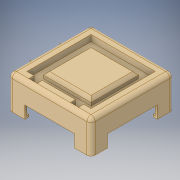
# Autodesk Inventor part: model for case
Saved by Autodesk Inventor 2016 (Build 200138000, 138)
## iProperties
Created: 2016-08-06
Part Number: model for case
Material: Polyethylene, High Density
Document SubType Name: Modeling
Designer: Jorian Brusind
Density: 0.952 g/cm^3
Appearance: Smooth - Off-White
Author: Jorian Brusind
Autodesk Inventor part; units mm, degrees
ref_plane "YZ Plane" through (0, 0, 0) normal (1, 0, 0) x (0, 1, 0)
ref_plane "XZ Plane" through (0, 0, 0) normal (0, 1, 0) x (-1, 0, 0)
ref_plane "XY Plane" through (0, 0, 0) normal (0, 0, 1) x (1, 0, 0)
sketch "Sketch4" plane through (0, 0, 0) normal (0, 1, 0) x (-1, 0, 0)
  line L0 (0, 0) -> (127, 0)
  line L1 (127, 0) -> (127, -127)
  line L2 (127, -127) -> (0, -127)
  line L3 (0, -127) -> (0, 0)
  dimension "d16" = 127
  dimension "d17" = 127
  constraints: 8 end point, 2 parallel, 1 horizontal, 1 perpendicular
  measures "d16" distance of L1.end L2.end
  measures "d17" distance of L0.end L1.end
extrude "Extrusion4" add sketch "Sketch4" along normal blind 50.8
sketch "Sketch5" plane through (0, 50.8, 0) normal (0, 1, 0) x (1, 0, 0)
  line L0 (0, 0) -> (0, 127) projected
  line L1 (-127, 127) -> (-127, 0) projected
  line L2 (-127, 0) -> (0, 0) projected
  line L3 (0, 127) -> (-127, 127) projected
  line L4 (0, 127) -> (0, 114.3)
  line L5 (-127, 0) -> (-127, 14.2875)
  line L6 (-112.6998, 14.2875) -> (-14.2748, 14.2875)
  line L7 (-14.2748, 14.2875) -> (-14.2748, 112.7125)
  line L8 (-14.2748, 112.7125) -> (-112.6998, 112.7125)
  line L9 (-112.6998, 112.7125) -> (-112.6998, 14.2875)
  line L10 (-112.6998, 14.2875) -> (-112.6998, 26.9875)
  line L11 (-99.9998, 26.9875) -> (-26.9748, 26.9875)
  line L12 (-14.2748, 14.2875) -> (-26.9748, 14.2875)
  line L13 (-26.9748, 26.9875) -> (-26.9748, 100.0125)
  line L14 (-112.6998, 112.7125) -> (-99.9998, 112.7125)
  line L15 (-99.9998, 100.0125) -> (-99.9998, 26.9875)
  line L16 (-112.6998, 112.7125) -> (-112.6998, 100.0125)
  line L17 (-99.9998, 100.0125) -> (-26.9748, 100.0125)
  dimension "d98" = 14.2875
  dimension "d99" = 112.7252
  dimension "d100" = 98.425
  dimension "d101" = 98.425
  dimension "d102" = 12.7
  dimension "d103" = 12.7
  dimension "d104" = 12.7
  dimension "d105" = 12.7
  dimension "d106" = 12.7
  dimension "d107" = 12.7
  dimension "d108" = 12.7
  dimension "d109" = 12.7
  dimension "d110" = 14.3002
  constraints: 28 end point, 8 perpendicular, 6 point on line
  measures "d98" distance of L1.end L5.end
  measures "d99" distance of L5.end L6.end
  measures "d100" distance of L6.end L7.end
  measures "d101" distance of L7.end L8.end
  measures "d102" distance of L6.start L10.end
  measures "d103" distance of L6.end L12.end
  measures "d104" distance of L8.end L14.end
  measures "d105" distance of L8.end L16.end
  measures "d106" distance between parallel lines of L9 L15
  measures "d107" distance between parallel lines of L7 L13
  measures "d108" distance between parallel lines of L8 L17
  measures "d109" distance between parallel lines of L6 L11
  measures "d110" distance between parallel lines of L1 L9
sketch "Sketch13" plane through (0, 50.8, 0) normal (0, 1, 0) x (1, 0, 0)
  line L0 (-127, 127) -> (-127, 0) projected
  line L1 (-127, 0) -> (-88.9, 0)
  line L2 (0, 127) -> (0, 0) projected
  line L3 (0, 0) -> (-38.1, 0)
  line L4 (-127, 0) -> (0, 0) projected
  line L5 (-88.9, 0) -> (-88.9, 14.3002)
  line L6 (-38.1, 0) -> (-38.1, 14.3002)
  line L7 (-88.9, 14.3002) -> (-101.6, 14.3002)
  line L8 (-101.6, 14.3002) -> (-101.6, 6.35)
  line L9 (-101.6, 6.35) -> (-88.9, 6.35)
  line L10 (-88.9, 6.35) -> (-88.9, 14.3002)
  line L11 (-38.1, 14.3002) -> (-25.4, 14.3002)
  line L12 (-25.4, 14.3002) -> (-25.4, 6.35)
  line L13 (-25.4, 6.35) -> (-38.1, 6.35)
  line L14 (-38.1, 6.35) -> (-38.1, 14.3002)
  dimension "d65" = 38.1
  dimension "d66" = 38.1
  dimension "d67" = 12.7
  dimension "d68" = 7.9502
  dimension "d69" = 12.7
  dimension "d70" = 7.9502
  dimension "d113" = 6.35
  dimension "d114" = 6.35
  constraints: 24 end point, 5 parallel, 3 horizontal, 2 perpendicular, 1 point on line, 1 vertical
  measures "d65" distance of L0.end L1.end
  measures "d66" distance of L2.end L3.end
  measures "d67" distance of L9.end L8.end
  measures "d68" distance of L8.end L7.end
  measures "d69" distance of L12.end L13.end
  measures "d70" distance of L11.end L12.end
  measures "d113" distance between parallel lines of L4 L13
  measures "d114" distance between parallel lines of L4 L9
extrude "Extrusion11" cut sketch "Sketch13" against normal blind 25.4
extrude "Extrusion13" cut sketch "Sketch5" against normal blind 9.525 contours L9 L8 L7 L6
chamfer "Chamfer1" distance 4.7625 angle 45 4 edges at (-63.4873, 50.8, -100.0125) (-99.9998, 50.8, -63.5) (-63.4873, 50.8, -26.9875) (-26.9748, 50.8, -63.5)
shell "Shell1" thickness 3.175 removed faces 0
sketch "Sketch16" plane through (0, 0, 0) normal (0, -1, 0) x (1, 0, 0)
  line L0 (-127, 0) -> (0, 0) projected
  line L1 (-127, 0) -> (-101.6, 0)
  line L2 (-88.9, -6.35) -> (-101.6, -6.35) projected
  line L3 (-101.6, 0) -> (-101.6, -6.35)
  line L4 (-101.6, -6.35) -> (-120.65, -6.35)
  line L5 (-120.65, -6.35) -> (-120.65, -25.4)
  line L6 (-120.65, -25.4) -> (-127, -25.4)
  line L7 (-127, -25.4) -> (-127, 0)
  line L8 (0, 0) -> (-25.4, 0)
  line L9 (-25.4, 0) -> (-25.4, -6.35)
  line L10 (-25.4, -6.35) -> (-6.35, -6.35)
  line L11 (-6.35, -6.35) -> (-6.35, -25.4)
  line L12 (-6.35, -25.4) -> (0, -25.4)
  line L13 (0, 0) -> (0, -127) projected
  line L14 (0, -25.4) -> (0, 0)
  line L15 (-127, -127) -> (-127, 0) projected
  line L16 (-127, -127) -> (-101.6, -127)
  line L17 (-101.6, -127) -> (-101.6, -120.65)
  line L18 (-101.6, -120.65) -> (-120.65, -120.65)
  line L19 (-120.65, -120.65) -> (-120.65, -101.6)
  line L20 (-120.65, -101.6) -> (-127, -101.6)
  line L21 (-127, -127) -> (-127, -101.6)
  line L22 (0, -127) -> (-25.4, -127)
  line L23 (-25.4, -127) -> (-25.4, -120.65)
  line L24 (-25.4, -120.65) -> (-6.35, -120.65)
  line L25 (-6.35, -120.65) -> (-6.35, -101.6)
  line L26 (-6.35, -101.6) -> (0, -101.6)
  line L27 (0, -101.6) -> (0, -127)
  line L28 (-127, -127) -> (0, -127)
  line L29 (0, -127) -> (0, 0)
  line L30 (0, 0) -> (-127, 0)
  line L31 (-127, 0) -> (-127, -127)
  dimension "d148" = 25.4
  dimension "d149" = 19.05
  dimension "d150" = 19.05
  dimension "d151" = 25.4
  dimension "d152" = 6.35
  dimension "d153" = 19.05
  dimension "d154" = 19.05
  dimension "d155" = 25.4
  dimension "d156" = 6.35
  dimension "d157" = 19.05
  dimension "d158" = 6.35
  dimension "d159" = 25.4
  dimension "d160" = 6.35
  dimension "d161" = 19.05
  dimension "d162" = 25.4
  constraints: 56 end point, 17 perpendicular, 4 point on line, 3 horizontal, 3 vertical, 2 parallel
  measures "d148" distance of L0.start L1.end
  measures "d149" distance of L2.end L4.end
  measures "d150" distance of L4.end L5.end
  measures "d151" distance of L0.end L8.end
  measures "d152" distance of L8.end L9.end
  measures "d153" distance of L9.end L10.end
  measures "d154" distance of L10.end L11.end
  measures "d155" distance of L15.start L16.end
  measures "d156" distance of L16.end L17.end
  measures "d157" distance of L18.end L19.end
  measures "d158" distance of L19.end L20.end
  measures "d159" distance of L13.end L22.end
  measures "d160" distance of L25.end L26.end
  measures "d161" distance of L24.end L25.end
  measures "d162" distance of L26.end L13.end
extrude "Extrusion15" cut sketch "Sketch16" against normal blind 19.05 contours L0 L9 L10 L11 L12 L13 L26 L25 L24 L23 L28 L17 L18 L19 L20 L15 L6 L5 L4 L3
fillet "Fillet1" radius 6.35 8 edges at (0, 25.4, 0) (0, 25.4, -127) (-127, 25.4, 0) (-127, 25.4, -127) (-127, 50.8, -63.5) (-63.5, 50.8, 0) (-63.5, 50.8, -127) (0, 50.8, -63.5)
sketch "Sketch24" plane through (-127, 0, -101.6) normal (-1, 0, 0) x (0, 0, 1)
  line L0 (101.6, 0) -> (101.6, 47.625)
  line L1 (101.6, 47.625) -> (63.5, 47.625)
  line L2 (63.5, 47.625) -> (63.5, 25.4)
  line L3 (63.5, 47.625) -> (63.5, 43.6563)
  circle A0 centre (63.5, 43.6563) radius 1.5875
  line L4 (63.5, 25.4) -> (63.5, 29.3688)
  circle A1 centre (63.5, 29.3688) radius 1.5875
  line L5 (63.5, 43.6563) -> (19.05, 43.6563)
  line L6 (63.5, 29.3688) -> (19.05, 29.3688)
  circle A2 centre (19.05, 43.6563) radius 1.5875
  circle A3 centre (19.05, 29.3688) radius 1.5875
  dimension "d206" = 47.625
  dimension "d207" = 38.1
  dimension "d208" = 22.225
  dimension "d209" = 3.9688
  dimension "d210" = 3.175
  dimension "d211" = 3.9688
  dimension "d212" = 3.175
  dimension "d213" = 44.45
  dimension "d214" = 44.45
  dimension "d215" = 3.175
  dimension "d216" = 3.175
  constraints: 14 end point, 4 centre point, 4 coincident, 3 horizontal, 2 point on line, 1 perpendicular, 1 vertical
  measures "d206" distance of L0.start L0.end
  measures "d207" distance of L0.end L1.end
  measures "d208" distance of L1.end L2.end
  measures "d209" distance of L1.end L3.end
  measures "d210" diameter of A0
  measures "d211" distance of L2.end L4.end
  measures "d212" diameter of A1
  measures "d213" distance of L5.start L5.end
  measures "d214" distance of L6.start L6.end
  measures "d215" diameter of A2
  measures "d216" diameter of A3
extrude "Extrusion23" add sketch "Sketch24" along normal blind 3.175
body "Solid2"
